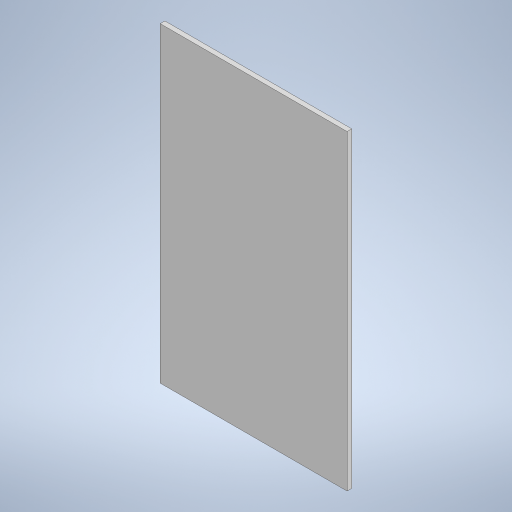
# Autodesk Inventor part: arcade kast 3d
Saved by Autodesk Inventor 2024 (Build 280153000, 153)
## iProperties
Created: 2024-03-18
Part Number: arcade kast 3d
Material: Generic
Document SubType Name: Modeling
Designer: domie
Density: 1 g/cm^3
Appearance: Default
Author: domie
Autodesk Inventor part; units mm, degrees
ref_plane "YZ Plane" through (0, 0, 0) normal (1, 0, 0) x (0, 1, 0)
ref_plane "XZ Plane" through (0, 0, 0) normal (0, 1, 0) x (-1, 0, 0)
ref_plane "XY Plane" through (0, 0, 0) normal (0, 0, 1) x (1, 0, 0)
sketch "Sketch1" plane through (0, 0, 0) normal (0, 0, 1) x (1, 0, 0)
  line L0 (-300, 500) -> (300, 500)
  line L1 (300, 500) -> (300, -500)
  line L2 (300, -500) -> (-300, -500)
  line L3 (-300, -500) -> (-300, 500)
  line L4 (-300, 500) -> (300, -500) construction
  line L5 (300, 500) -> (-300, -500) construction
  point P0 (0, 0)
  dimension "d0" = 1000
  dimension "d1" = 600
  constraints: 12 end point, 2 midpoint, 2 parallel, 1 horizontal, 1 perpendicular
  measures "d0" distance of L0.end L1.end
  measures "d1" distance of L1.end L2.end
extrude "achterkant onder" add sketch "Sketch1" along normal blind 15
sketch "Sketch2" plane through (300, -500, 0) normal (1, 0, 0) x (0, 0, -1)
  line L0 (0, 0) -> (-400, 0)
  line L1 (0, 0) -> (0, 1000) projected
  line L2 (0, 1000) -> (-500, 1000)
  line L3 (-500, 1000) -> (-400, 0)
  point P0 (0, 500)
  dimension "d4" = 400
  dimension "d5" = 500
  constraints: 6 end point, 2 horizontal
  measures "d4" distance of L0.start L0.end
  measures "d5" distance of L1.end L2.end
extrude "Extrusion2" [suppressed]
sketch "Sketch3" plane through (-300, -500, 0) normal (-1, 0, 0) x (0, 0, 1)
  line L0 (15, 1100) -> (500, 1100) projected
  line L1 (0, 1100) -> (500, 1100)
  line L2 (500, 1100) -> (400, 0) projected
  line L3 (500, 1100) -> (400, 0)
  line L4 (400, 0) -> (0, 0)
  line L5 (0, 0) -> (0, 1100)
  point P0 (0, 500)
  point P1 (15, 1000)
  point P2 (15, 1100)
  constraints: 8 end point, 2 horizontal, 1 collinear, 1 perpendicular, 1 other
extrude "Extrusion3" [suppressed]
sketch "Sketch4" plane through (-300, -550, 400) normal (0, -0.0905357, 0.9958932) x (1, 0, 0)
  line L0 (600, 1104.5361) -> (615, 1104.5361) projected
  line L1 (-15.8911, 1104.5361) -> (615, 1104.5361)
  line L2 (600, 0) -> (615, 0) projected
  line L3 (615, 1104.5361) -> (615, 0)
  line L4 (615, 0) -> (-15.8911, 0)
  line L5 (-15.8911, 0) -> (-15.8911, 1104.5361)
  line L6 (-15.8911, 1104.5361) -> (-15.8911, 0)
  point P0 (300, 511.527)
  constraints: 10 end point, 3 perpendicular, 1 horizontal, 1 vertical
extrude "Extrusion4" [suppressed]
sketch "Sketch5" plane through (-315, 550, 0) normal (0, 1, 0) x (1, 0, 0)
  line L0 (615, -500) -> (15, -500) projected
  line L1 (15, -500) -> (615, -500)
  line L2 (615, -500) -> (615, -300)
  line L3 (615, -300) -> (15, -300)
  line L4 (15, -300) -> (15, -500)
  point P0 (315, 0)
  dimension "d12" = 221.503
  constraints: 8 end point, 2 parallel, 1 horizontal, 1 perpendicular
extrude "Extrusion5" [suppressed]
sketch "Sketch6" plane through (-315, 550, 0) normal (0, 1, 0) x (1, 0, 0)
  line L0 (0, 0) -> (630, 0) projected
  line L1 (630, 0) -> (0, 0)
  line L2 (0, 0) -> (0, -15)
  line L3 (0, -15) -> (630, -15)
  line L4 (630, 0) -> (630, -500) projected
  line L5 (630, -15) -> (630, 0)
  point P0 (315, 0)
  dimension "d15" = 15
  constraints: 8 end point, 2 perpendicular, 1 collinear, 1 horizontal
  measures "d15" distance of L0.start L2.end
extrude "Extrusion6" [suppressed]
sketch "Sketch7" plane through (-315, 550, 500) normal (0, 1, 0) x (1, 0, 0)
  line L0 (0, 485) -> (630, 485) projected
  line L1 (615, 200) -> (15, 200) projected
  line L2 (630, 485) -> (615, 485)
  line L3 (615, 485) -> (615, 200)
  line L4 (615, 200) -> (630, 200)
  line L5 (630, 200) -> (630, 485)
  line L6 (15, 485) -> (15, 100) projected
  line L7 (0, 500) -> (0, 100) projected
  line L8 (15, 485) -> (0, 485)
  line L9 (0, 485) -> (0, 200)
  line L10 (0, 200) -> (15, 200)
  line L11 (15, 200) -> (15, 485)
  point P0 (315, 500)
  constraints: 16 end point, 4 parallel, 2 horizontal, 2 perpendicular, 2 point on line
extrude "Extrusion7" [suppressed]
sketch "Sketch10" plane through (-315, -550, 0) normal (-1, 0, 0) x (0, 0, 1)
  line L0 (0, 1700) -> (300, 1700) projected
  line L1 (300, 1700) -> (300, 1800)
  line L2 (300, 1800) -> (0, 1700)
  line L3 (0, 1700) -> (300, 1700)
  point P0 (0, 550)
  dimension "d24" = 100
  constraints: 6 end point, 1 collinear, 1 vertical
  measures "d24" distance of L0.end L1.end
extrude "Extrusion10" [suppressed]
sketch "Sketch11" plane through (300, -550, 0) normal (-1, 0, 0) x (0, 0, 1)
  line L0 (300, 1700) -> (300, 1800)
  line L1 (300, 1800) -> (0, 1700)
  line L2 (300, 1700) -> (0, 1700) projected
  line L3 (0, 1700) -> (300, 1700)
  point P0 (0, 550)
  dimension "d27" = 100
  constraints: 6 end point, 1 collinear, 1 vertical
  measures "d27" distance of L0.start L0.end
extrude "Extrusion11" [suppressed]
sketch "Sketch12" plane through (300, 1250, 300) normal (0, 0.9486833, -0.3162278) x (1, 0, 0)
  line L0 (15, 221.3594) -> (15, 0) projected
  line L1 (-615, 221.3594) -> (-615, 0) projected
  line L2 (15, 0) -> (-615, 0)
  line L3 (-600, 316.2278) -> (-615, 316.2278) projected
  line L4 (-615, 0) -> (-615, 316.2278)
  line L5 (-615, 316.2278) -> (15, 316.2278)
  line L6 (15, 316.2278) -> (15, 0)
  point P0 (-300, 679.8897)
  point P1 (-600, 316.2278)
  constraints: 8 end point, 3 perpendicular, 1 horizontal
extrude "Extrusion12" [suppressed]
body "Solid1"
